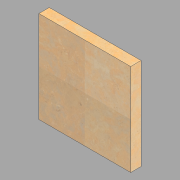
# Autodesk Inventor part: 8-1x-17.625x17.625x2 as paver
Saved by Autodesk Inventor 2022.1 (Build 261234020, 234B)
## iProperties
Created: 2021-11-03
Part Number: 8-1x-17.625x17.625x2 as paver
Material: Limestone
Document SubType Name: Modeling
Designer: awelt
Density: 2.6 g/cm^3
Appearance: Amber Select
Mass: 26470.5 g
Surface Area: 4917.93 cm^2
Volume: 10181 cm^3
Author: awelt
Autodesk Inventor part; units mm, degrees
ref_plane "YZ Plane" through (0, 0, 0) normal (1, 0, 0) x (0, 1, 0)
ref_plane "XZ Plane" through (0, 0, 0) normal (0, 1, 0) x (-1, 0, 0)
ref_plane "XY Plane" through (0, 0, 0) normal (0, 0, 1) x (1, 0, 0)
sketch "Sketch1" plane through (0, 0, 0) normal (0, 0, 1) x (1, 0, 0)
  line L0 (-223.8375, 223.8375) -> (223.8375, 223.8375)
  line L1 (223.8375, 223.8375) -> (223.8375, -223.8375)
  line L2 (223.8375, -223.8375) -> (-223.8375, -223.8375)
  line L3 (-223.8375, -223.8375) -> (-223.8375, 223.8375)
  line L4 (-223.8375, 223.8375) -> (223.8375, -223.8375) construction
  line L5 (223.8375, 223.8375) -> (-223.8375, -223.8375) construction
  point P0 (0, 0)
  dimension "d0" = 447.675
  dimension "d1" = 447.675
  constraints: 12 end point, 2 midpoint, 2 parallel, 1 horizontal, 1 perpendicular
  measures "d0" distance of L1.end L2.end
  measures "d1" distance of L0.end L1.end
extrude "Extrusion1" add sketch "Sketch1" along normal blind 50.8
body "Solid1"
